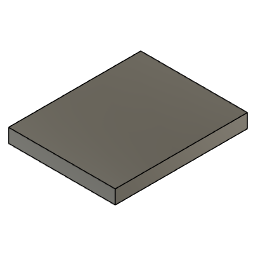
Mold Design Day#20 v4 (Autodesk Fusion 360 design; units mm, degrees)
Autodesk Fusion 360 part; units mm, degrees
box "BoxPrimitive1" add length 50 width 35 height 3 placed x (0, 1, 0) y (-1, 0, 0) z (0, 0, 1) at (35, 0, 0) makes body 1 in component "Keychaing"
fillet "Fillet1" radius 7 4 edges at (35, 0, 1.5) (0, 0, 1.5) (0, 50, 1.5) (35, 50, 1.5) on bodies 1 in component "Keychaing"
sketch "Sketch2" plane through (0, 0, 3) normal (0, 0, 1) x (-1, 0, 0) in component "Keychaing"
  arc A0 (-35, -43) -> (-28, -50) centre (-28, -43) ccw
  line L0 (-28, -50) -> (-7, -50)
  arc A1 (-7, -50) -> (0, -43) centre (-7, -43) ccw
  line L1 (0, -43) -> (0, -7)
  arc A2 (0, -7) -> (-7, 0) centre (-7, -7) ccw
  line L2 (-7, 0) -> (-28, 0)
  arc A3 (-28, 0) -> (-35, -7) centre (-28, -7) ccw
  line L3 (-35, -7) -> (-35, -43)
  line L4 (-17.5, -50) -> (-17.5, -45)
  dimension "d8" = 5
  constraint vertical L4
  constraint midpoint L0 L4.start
  measures "d8" distance of L4.start L4.end
hole "Hole1" at (17.5, 45, 3) direction (0, 0, -1) diameter 5 depth 3 tip angle 180 bodies 1 in component "Keychaing"
sketch "Sketch3" plane through (0, 0, 3) normal (0, 0, 1) x (-1, 0, 0) in component "Keychaing"
  circle A0 centre (-17.5, -45) radius 2.5
  arc A1 (-35, -43) -> (-28, -50) centre (-28, -43) ccw
  line L0 (-28, -50) -> (-7, -50)
  arc A2 (-7, -50) -> (0, -43) centre (-7, -43) ccw
  line L1 (0, -43) -> (0, -7)
  arc A3 (0, -7) -> (-7, 0) centre (-7, -7) ccw
  line L2 (-7, 0) -> (-28, 0)
  arc A4 (-28, 0) -> (-35, -7) centre (-28, -7) ccw
  line L3 (-35, -7) -> (-35, -43)
  spline S0 degree 3 poles (-7.2465, -28.2329) (-7.1727, -28.1591) (-7.1727, -22.1159) (-7.2465, -22.0421) knots 0 0 0 0 1 1 1 1
  spline S1 degree 3 poles (-7.2465, -22.0421) (-7.3203, -21.9683) (-8.9136, -21.9683) (-8.9614, -22.0465) knots 0 0 0 0 1 1 1 1
  spline S2 degree 3 poles (-8.9614, -22.0465) (-8.9787, -22.0725) (-9.0048, -22.6543) (-9.0178, -23.3358) knots 0 0 0 0 1 1 1 1
  line L4 (-9.0178, -23.3358) -> (-9.0395, -24.5731)
  line L5 (-9.0395, -24.5731) -> (-9.5561, -23.3575)
  spline S3 degree 3 poles (-9.5561, -23.3575) (-9.8383, -22.689) (-10.0988, -22.1072) (-10.1379, -22.0682) knots 0 0 0 0 1 1 1 1
  spline S4 degree 3 poles (-10.1379, -22.0682) (-10.1943, -21.9987) (-10.2985, -21.99) (-11.0409, -21.99) knots 0 0 0 0 1 1 1 1
  spline S5 degree 3 poles (-11.0409, -21.99) (-11.8744, -21.99) (-11.8831, -21.99) (-11.9482, -22.0942) knots 0 0 0 0 1 1 1 1
  spline S6 degree 3 poles (-11.9482, -22.0942) (-12.009, -22.181) (-12.0133, -22.5501) (-12.0046, -25.1983) knots 0 0 0 0 1 1 1 1
  spline S7 degree 3 poles (-12.0046, -25.1983) (-11.9916, -27.8118) (-11.9829, -28.2068) (-11.9265, -28.2416) knots 0 0 0 0 1 1 1 1
  spline S8 degree 3 poles (-11.9265, -28.2416) (-11.8223, -28.3067) (-10.2464, -28.298) (-10.203, -28.2329) knots 0 0 0 0 1 1 1 1
  spline S9 degree 3 poles (-10.203, -28.2329) (-10.1856, -28.2025) (-10.1596, -27.6207) (-10.1465, -26.9435) knots 0 0 0 0 1 1 1 1
  line L6 (-10.1465, -26.9435) -> (-10.1248, -25.7149)
  line L7 (-10.1248, -25.7149) -> (-9.5865, -26.9739)
  spline S10 degree 3 poles (-9.5865, -26.9739) (-9.2913, -27.6685) (-9.0221, -28.2459) (-8.9874, -28.2589) knots 0 0 0 0 1 1 1 1
  spline S11 degree 3 poles (-8.9874, -28.2589) (-8.8528, -28.311) (-7.2986, -28.285) (-7.2465, -28.2329) knots 0 0 0 0 1 1 1 1
  spline S12 degree 3 poles (-9.5171, -26.6092) (-10.0901, -25.2634) (-10.1683, -25.1115) (-10.2507, -25.1245) knots 0 0 0 0 1 1 1 1
  spline S13 degree 3 poles (-10.2507, -25.1245) (-10.3419, -25.1375) (-10.3419, -25.1418) (-10.3549, -26.6266) knots 0 0 0 0 1 1 1 1
  line L8 (-10.3549, -26.6266) -> (-10.3636, -28.1113)
  line L9 (-10.3636, -28.1113) -> (-11.0799, -28.1113)
  line L10 (-11.0799, -28.1113) -> (-11.7963, -28.1113)
  line L11 (-11.7963, -28.1113) -> (-11.7876, -25.1505)
  line L12 (-11.7876, -25.1505) -> (-11.7746, -22.1854)
  line L13 (-11.7746, -22.1854) -> (-11.0539, -22.1724)
  spline S14 degree 3 poles (-11.0539, -22.1724) (-10.5112, -22.1637) (-10.3202, -22.1767) (-10.2855, -22.2158) knots 0 0 0 0 1 1 1 1
  spline S15 degree 3 poles (-10.2855, -22.2158) (-10.2594, -22.2462) (-10.0424, -22.7411) (-9.7992, -23.3141) knots 0 0 0 0 1 1 1 1
  spline S16 degree 3 poles (-9.7992, -23.3141) (-9.0135, -25.1766) (-9.0178, -25.1635) (-8.9136, -25.1505) knots 0 0 0 0 1 1 1 1
  spline S17 degree 3 poles (-8.9136, -25.1505) (-8.8224, -25.1375) (-8.8224, -25.1288) (-8.8094, -23.6484) knots 0 0 0 0 1 1 1 1
  line L14 (-8.8094, -23.6484) -> (-8.8007, -22.1637)
  line L15 (-8.8007, -22.1637) -> (-8.0931, -22.1724)
  line L16 (-8.0931, -22.1724) -> (-7.3898, -22.1854)
  line L17 (-7.3898, -22.1854) -> (-7.3768, -25.0941)
  spline S18 degree 3 poles (-7.3768, -25.0941) (-7.3724, -26.696) (-7.3768, -28.0288) (-7.3898, -28.0592) knots 0 0 0 0 1 1 1 1
  spline S19 degree 3 poles (-7.3898, -28.0592) (-7.4028, -28.0983) (-7.5938, -28.1113) (-8.1452, -28.1113) knots 0 0 0 0 1 1 1 1
  line L18 (-8.1452, -28.1113) -> (-8.8789, -28.1113)
  line L19 (-8.8789, -28.1113) -> (-9.5171, -26.6092)
  spline S20 degree 3 poles (-13.8454, -28.2112) (-13.8237, -28.1678) (-13.446, -26.7872) (-13.0118, -25.1418) knots 0 0 0 0 1 1 1 1
  spline S21 degree 3 poles (-13.0118, -25.1418) (-12.4127, -22.8974) (-12.2261, -22.1333) (-12.2608, -22.0812) knots 0 0 0 0 1 1 1 1
  spline S22 degree 3 poles (-12.2608, -22.0812) (-12.2999, -22.0204) (-12.4214, -22.0117) (-13.1898, -22.0117) knots 0 0 0 0 1 1 1 1
  line L20 (-13.1898, -22.0117) -> (-14.0711, -22.0117)
  line L21 (-14.0711, -22.0117) -> (-14.1276, -22.1637)
  spline S23 degree 3 poles (-14.1276, -22.1637) (-14.1536, -22.2462) (-14.2014, -22.4285) (-14.2274, -22.5674) knots 0 0 0 0 1 1 1 1
  line L22 (-14.2274, -22.5674) -> (-14.2795, -22.8192)
  line L23 (-14.2795, -22.8192) -> (-14.8916, -22.8062)
  line L24 (-14.8916, -22.8062) -> (-15.5038, -22.7932)
  line L25 (-15.5038, -22.7932) -> (-15.5819, -22.4502)
  spline S24 degree 3 poles (-15.5819, -22.4502) (-15.6253, -22.2592) (-15.6818, -22.0812) (-15.7122, -22.0465) knots 0 0 0 0 1 1 1 1
  spline S25 degree 3 poles (-15.7122, -22.0465) (-15.7469, -21.9987) (-15.9379, -21.99) (-16.6282, -21.9987) knots 0 0 0 0 1 1 1 1
  spline S26 degree 3 poles (-16.6282, -21.9987) (-17.3836, -22.0117) (-17.5008, -22.0204) (-17.5399, -22.0855) knots 0 0 0 0 1 1 1 1
  spline S27 degree 3 poles (-17.5399, -22.0855) (-17.5746, -22.1376) (-17.4009, -22.867) (-16.7931, -25.1679) knots 0 0 0 0 1 1 1 1
  spline S28 degree 3 poles (-16.7931, -25.1679) (-16.3547, -26.8219) (-15.977, -28.2025) (-15.9553, -28.2329) knots 0 0 0 0 1 1 1 1
  spline S29 degree 3 poles (-15.9553, -28.2329) (-15.9205, -28.2719) (-15.6557, -28.285) (-14.896, -28.285) knots 0 0 0 0 1 1 1 1
  spline S30 degree 3 poles (-14.896, -28.285) (-13.9756, -28.285) (-13.8801, -28.2763) (-13.8454, -28.2112) knots 0 0 0 0 1 1 1 1
  spline S31 degree 3 poles (-16.5544, -25.2504) (-16.9668, -23.6918) (-17.3184, -22.359) (-17.3315, -22.2896) knots 0 0 0 0 1 1 1 1
  line L26 (-17.3315, -22.2896) -> (-17.3619, -22.1637)
  line L27 (-17.3619, -22.1637) -> (-16.6499, -22.1637)
  spline S32 degree 3 poles (-16.6499, -22.1637) (-16.2592, -22.1637) (-15.9205, -22.181) (-15.8945, -22.1984) knots 0 0 0 0 1 1 1 1
  spline S33 degree 3 poles (-15.8945, -22.1984) (-15.8684, -22.2158) (-15.8207, -22.3373) (-15.7946, -22.4676) knots 0 0 0 0 1 1 1 1
  spline S34 degree 3 poles (-15.7946, -22.4676) (-15.7642, -22.5978) (-15.7208, -22.7715) (-15.6948, -22.8496) knots 0 0 0 0 1 1 1 1
  line L28 (-15.6948, -22.8496) -> (-15.6514, -22.9885)
  line L29 (-15.6514, -22.9885) -> (-14.9003, -22.9885)
  spline S35 degree 3 poles (-14.9003, -22.9885) (-14.0364, -22.9885) (-14.1015, -23.0233) (-14.0103, -22.5544) knots 0 0 0 0 1 1 1 1
  spline S36 degree 3 poles (-14.0103, -22.5544) (-13.98, -22.3981) (-13.9365, -22.2462) (-13.9105, -22.2201) knots 0 0 0 0 1 1 1 1
  spline S37 degree 3 poles (-13.9105, -22.2201) (-13.8801, -22.1767) (-13.6761, -22.1637) (-13.1551, -22.1637) knots 0 0 0 0 1 1 1 1
  line L30 (-13.1551, -22.1637) -> (-12.4388, -22.1637)
  line L31 (-12.4388, -22.1637) -> (-12.4692, -22.2852)
  spline S38 degree 3 poles (-12.4692, -22.2852) (-12.5126, -22.4719) (-13.9669, -27.9507) (-13.993, -28.0375) knots 0 0 0 0 1 1 1 1
  spline S39 degree 3 poles (-13.993, -28.0375) (-14.0147, -28.107) (-14.0885, -28.1113) (-14.9133, -28.1026) knots 0 0 0 0 1 1 1 1
  line L32 (-14.9133, -28.1026) -> (-15.8077, -28.0896)
  line L33 (-15.8077, -28.0896) -> (-16.5544, -25.2504)
  spline S40 degree 3 poles (-14.7961, -26.1447) (-14.731, -26.0622) (-14.3403, -24.2215) (-14.375, -24.139) knots 0 0 0 0 1 1 1 1
  spline S41 degree 3 poles (-14.375, -24.139) (-14.4097, -24.0391) (-15.3475, -24.0435) (-15.3866, -24.1433) knots 0 0 0 0 1 1 1 1
  spline S42 degree 3 poles (-15.3866, -24.1433) (-15.4169, -24.2215) (-15.0696, -25.9276) (-14.9915, -26.0796) knots 0 0 0 0 1 1 1 1
  spline S43 degree 3 poles (-14.9915, -26.0796) (-14.9307, -26.1968) (-14.8612, -26.2228) (-14.7961, -26.1447) knots 0 0 0 0 1 1 1 1
  spline S44 degree 3 poles (-15.1825, -24.304) (-15.1825, -24.2432) (-14.6398, -24.2215) (-14.6051, -24.2823) knots 0 0 0 0 1 1 1 1
  spline S45 degree 3 poles (-14.6051, -24.2823) (-14.5834, -24.3126) (-14.8135, -25.4674) (-14.8656, -25.5933) knots 0 0 0 0 1 1 1 1
  spline S46 degree 3 poles (-14.8656, -25.5933) (-14.8873, -25.6498) (-15.1782, -24.4646) (-15.1825, -24.304) knots 0 0 0 0 1 1 1 1
  spline S47 degree 3 poles (-17.8828, -28.2329) (-17.809, -28.1591) (-17.809, -22.1159) (-17.8828, -22.0421) knots 0 0 0 0 1 1 1 1
  spline S48 degree 3 poles (-17.8828, -22.0421) (-17.9219, -22.0031) (-18.2866, -21.99) (-19.259, -21.99) knots 0 0 0 0 1 1 1 1
  spline S49 degree 3 poles (-19.259, -21.99) (-20.7481, -21.9944) (-20.9044, -22.0161) (-21.4254, -22.2766) knots 0 0 0 0 1 1 1 1
  spline S50 degree 3 poles (-21.4254, -22.2766) (-21.7857, -22.4589) (-22.0028, -22.6803) (-22.1677, -23.0276) knots 0 0 0 0 1 1 1 1
  spline S51 degree 3 poles (-22.1677, -23.0276) (-22.2719, -23.249) (-22.2806, -23.3185) (-22.2806, -23.8134) knots 0 0 0 0 1 1 1 1
  spline S52 degree 3 poles (-22.2806, -23.8134) (-22.2806, -24.317) (-22.2719, -24.3734) (-22.159, -24.6165) knots 0 0 0 0 1 1 1 1
  spline S53 degree 3 poles (-22.159, -24.6165) (-22.0939, -24.7598) (-21.9593, -24.9595) (-21.8595, -25.0594) knots 0 0 0 0 1 1 1 1
  line L34 (-21.8595, -25.0594) -> (-21.6815, -25.2417)
  line L35 (-21.6815, -25.2417) -> (-21.8595, -25.4414)
  spline S54 degree 3 poles (-21.8595, -25.4414) (-22.3761, -26.0275) (-22.3153, -27.1996) (-21.7423, -27.7553) knots 0 0 0 0 1 1 1 1
  spline S55 degree 3 poles (-21.7423, -27.7553) (-21.5252, -27.9637) (-21.1605, -28.1417) (-20.7915, -28.2242) knots 0 0 0 0 1 1 1 1
  spline S56 degree 3 poles (-20.7915, -28.2242) (-20.4051, -28.3023) (-17.961, -28.311) (-17.8828, -28.2329) knots 0 0 0 0 1 1 1 1
  spline S57 degree 3 poles (-20.8393, -28.0115) (-21.6164, -27.7857) (-21.955, -27.3776) (-21.9897, -26.6092) knots 0 0 0 0 1 1 1 1
  spline S58 degree 3 poles (-21.9897, -26.6092) (-22.0158, -26.0709) (-21.9333, -25.8278) (-21.6164, -25.4978) knots 0 0 0 0 1 1 1 1
  line L36 (-21.6164, -25.4978) -> (-21.3819, -25.2504)
  line L37 (-21.3819, -25.2504) -> (-21.6164, -25.0159)
  spline S59 degree 3 poles (-21.6164, -25.0159) (-21.8899, -24.7468) (-22.0201, -24.4993) (-22.0896, -24.1346) knots 0 0 0 0 1 1 1 1
  spline S60 degree 3 poles (-22.0896, -24.1346) (-22.2285, -23.3966) (-21.9203, -22.7367) (-21.2951, -22.4372) knots 0 0 0 0 1 1 1 1
  spline S61 degree 3 poles (-21.2951, -22.4372) (-20.8176, -22.2071) (-20.6613, -22.1854) (-19.2851, -22.1854) knots 0 0 0 0 1 1 1 1
  line L38 (-19.2851, -22.1854) -> (-18.0261, -22.1854)
  line L39 (-18.0261, -22.1854) -> (-18.0131, -25.1505)
  line L40 (-18.0131, -25.1505) -> (-18.0044, -28.12)
  line L41 (-18.0044, -28.12) -> (-19.2938, -28.0983)
  spline S62 degree 3 poles (-19.2938, -28.0983) (-20.3183, -28.0853) (-20.6396, -28.0679) (-20.8393, -28.0115) knots 0 0 0 0 1 1 1 1
  spline S63 degree 3 poles (-19.5021, -26.8436) (-19.4891, -26.8089) (-19.4848, -26.5484) (-19.4891, -26.2619) knots 0 0 0 0 1 1 1 1
  line L42 (-19.4891, -26.2619) -> (-19.5021, -25.7453)
  line L43 (-19.5021, -25.7453) -> (-19.8147, -25.7323)
  spline S64 degree 3 poles (-19.8147, -25.7323) (-20.327, -25.7106) (-20.5527, -25.8625) (-20.5962, -26.2619) knots 0 0 0 0 1 1 1 1
  spline S65 degree 3 poles (-20.5962, -26.2619) (-20.6222, -26.479) (-20.531, -26.7134) (-20.3834, -26.8046) knots 0 0 0 0 1 1 1 1
  spline S66 degree 3 poles (-20.3834, -26.8046) (-20.2402, -26.8957) (-19.5325, -26.9261) (-19.5021, -26.8436) knots 0 0 0 0 1 1 1 1
  spline S67 degree 3 poles (-20.3053, -26.5832) (-20.3617, -26.518) (-20.3921, -26.4312) (-20.3921, -26.3053) knots 0 0 0 0 1 1 1 1
  spline S68 degree 3 poles (-20.3921, -26.3053) (-20.3921, -26.0448) (-20.2532, -25.9406) (-19.9102, -25.9406) knots 0 0 0 0 1 1 1 1
  line L44 (-19.9102, -25.9406) -> (-19.6541, -25.9406)
  line L45 (-19.6541, -25.9406) -> (-19.6541, -26.3097)
  line L46 (-19.6541, -26.3097) -> (-19.6541, -26.6787)
  line L47 (-19.6541, -26.6787) -> (-19.9363, -26.6787)
  spline S69 degree 3 poles (-19.9363, -26.6787) (-20.1664, -26.6787) (-20.2315, -26.6613) (-20.3053, -26.5832) knots 0 0 0 0 1 1 1 1
  spline S70 degree 3 poles (-19.5325, -24.6469) (-19.4935, -24.6165) (-19.4804, -24.4603) (-19.4891, -24.0044) knots 0 0 0 0 1 1 1 1
  line L48 (-19.4891, -24.0044) -> (-19.5021, -23.401)
  line L49 (-19.5021, -23.401) -> (-19.806, -23.3879)
  spline S71 degree 3 poles (-19.806, -23.3879) (-20.1924, -23.3706) (-20.3965, -23.4314) (-20.5441, -23.605) knots 0 0 0 0 1 1 1 1
  spline S72 degree 3 poles (-20.5441, -23.605) (-20.6526, -23.7309) (-20.6613, -23.77) (-20.6439, -24.0565) knots 0 0 0 0 1 1 1 1
  spline S73 degree 3 poles (-20.6439, -24.0565) (-20.6266, -24.4038) (-20.5614, -24.521) (-20.3183, -24.6209) knots 0 0 0 0 1 1 1 1
  spline S74 degree 3 poles (-20.3183, -24.6209) (-20.1664, -24.686) (-19.6237, -24.7034) (-19.5325, -24.6469) knots 0 0 0 0 1 1 1 1
  spline S75 degree 3 poles (-20.3357, -24.3604) (-20.4399, -24.2692) (-20.4572, -24.2215) (-20.4572, -24.0305) knots 0 0 0 0 1 1 1 1
  spline S76 degree 3 poles (-20.4572, -24.0305) (-20.4572, -23.8394) (-20.4399, -23.7917) (-20.3357, -23.7005) knots 0 0 0 0 1 1 1 1
  spline S77 degree 3 poles (-20.3357, -23.7005) (-20.2358, -23.6137) (-20.1664, -23.5963) (-19.9319, -23.5963) knots 0 0 0 0 1 1 1 1
  line L50 (-19.9319, -23.5963) -> (-19.6541, -23.5963)
  line L51 (-19.6541, -23.5963) -> (-19.6541, -24.0305)
  line L52 (-19.6541, -24.0305) -> (-19.6541, -24.4646)
  line L53 (-19.6541, -24.4646) -> (-19.9319, -24.4646)
  spline S78 degree 3 poles (-19.9319, -24.4646) (-20.1664, -24.4646) (-20.2358, -24.4472) (-20.3357, -24.3604) knots 0 0 0 0 1 1 1 1
  spline S79 degree 3 poles (-22.7017, -28.2329) (-22.6279, -28.1591) (-22.6279, -22.1159) (-22.7017, -22.0421) knots 0 0 0 0 1 1 1 1
  spline S80 degree 3 poles (-22.7017, -22.0421) (-22.7364, -22.0074) (-22.9926, -21.99) (-23.5613, -21.99) knots 0 0 0 0 1 1 1 1
  spline S81 degree 3 poles (-23.5613, -21.99) (-24.13, -21.99) (-24.3862, -22.0074) (-24.4209, -22.0421) knots 0 0 0 0 1 1 1 1
  spline S82 degree 3 poles (-24.4209, -22.0421) (-24.4947, -22.1159) (-24.4947, -28.1591) (-24.4209, -28.2329) knots 0 0 0 0 1 1 1 1
  spline S83 degree 3 poles (-24.4209, -28.2329) (-24.3471, -28.3067) (-22.7755, -28.3067) (-22.7017, -28.2329) knots 0 0 0 0 1 1 1 1
  line L54 (-24.2559, -25.1375) -> (-24.2559, -22.1637)
  line L55 (-24.2559, -22.1637) -> (-23.5526, -22.1724)
  line L56 (-23.5526, -22.1724) -> (-22.845, -22.1854)
  line L57 (-22.845, -22.1854) -> (-22.832, -25.0941)
  spline S84 degree 3 poles (-22.832, -25.0941) (-22.8276, -26.696) (-22.832, -28.0288) (-22.845, -28.0592) knots 0 0 0 0 1 1 1 1
  spline S85 degree 3 poles (-22.845, -28.0592) (-22.858, -28.0983) (-23.0447, -28.1113) (-23.5613, -28.1113) knots 0 0 0 0 1 1 1 1
  line L58 (-23.5613, -28.1113) -> (-24.2559, -28.1113)
  line L59 (-24.2559, -28.1113) -> (-24.2559, -25.1375)
  spline S86 degree 3 poles (-24.9158, -28.2329) (-24.842, -28.1591) (-24.842, -22.1159) (-24.9158, -22.0421) knots 0 0 0 0 1 1 1 1
  spline S87 degree 3 poles (-24.9158, -22.0421) (-24.9549, -22.0031) (-25.4715, -21.99) (-26.9779, -21.99) knots 0 0 0 0 1 1 1 1
  spline S88 degree 3 poles (-26.9779, -21.99) (-28.9185, -21.99) (-28.988, -21.9944) (-29.0314, -22.0725) knots 0 0 0 0 1 1 1 1
  spline S89 degree 3 poles (-29.0314, -22.0725) (-29.0531, -22.1203) (-29.0748, -22.4415) (-29.0748, -22.8105) knots 0 0 0 0 1 1 1 1
  spline S90 degree 3 poles (-29.0748, -22.8105) (-29.0748, -23.4357) (-29.0705, -23.4661) (-28.9793, -23.5269) knots 0 0 0 0 1 1 1 1
  spline S91 degree 3 poles (-28.9793, -23.5269) (-28.8968, -23.5876) (-28.7058, -23.5963) (-27.7854, -23.5963) knots 0 0 0 0 1 1 1 1
  line L60 (-27.7854, -23.5963) -> (-26.6871, -23.5963)
  line L61 (-26.6871, -23.5963) -> (-26.6871, -25.8886)
  spline S92 degree 3 poles (-26.6871, -25.8886) (-26.6871, -27.6121) (-26.674, -28.1938) (-26.635, -28.2329) knots 0 0 0 0 1 1 1 1
  spline S93 degree 3 poles (-26.635, -28.2329) (-26.5612, -28.3067) (-24.9896, -28.3067) (-24.9158, -28.2329) knots 0 0 0 0 1 1 1 1
  line L62 (-26.5134, -25.7453) -> (-26.5351, -23.401)
  line L63 (-26.5351, -23.401) -> (-27.6986, -23.3879)
  line L64 (-27.6986, -23.3879) -> (-28.8577, -23.3793)
  line L65 (-28.8577, -23.3793) -> (-28.8577, -22.7715)
  line L66 (-28.8577, -22.7715) -> (-28.8577, -22.1637)
  line L67 (-28.8577, -22.1637) -> (-26.9606, -22.1724)
  line L68 (-26.9606, -22.1724) -> (-25.0591, -22.1854)
  line L69 (-25.0591, -22.1854) -> (-25.046, -25.1505)
  line L70 (-25.046, -25.1505) -> (-25.0374, -28.1113)
  line L71 (-25.0374, -28.1113) -> (-25.7624, -28.1026)
  line L72 (-25.7624, -28.1026) -> (-26.4917, -28.0896)
  line L73 (-26.4917, -28.0896) -> (-26.5134, -25.7453)
extrude "Extrude1" add sketch "Sketch3" along normal blind 1 contours S12 S13 L8 L9 L10 L11 L12 L13 S14 S15 S16 S17 L14 L15 L16 L17 S18 S19 L18 L19 | S31 L26 L27 S32 S33 S34 L28 L29 S35 S36 S37 L30 L31 S38 S39 L32 L33 | S57 S58 L36 L37 S59 S60 S61 L38 L39 L40 L41 S62 | L54 L55 L56 L57 S84 S85 L58 L59 | L62 L63 L64 L65 L66 L67 L68 L69 L70 L71 L72 L73 bodies 1 in component "Keychaing"
box "BoxPrimitive2" add length 57 width 46 height 6 placed x (0, -1, 0) y (1, 0, 0) z (0, 0, 1) at (-5, 53, 0) separate body makes body 2 in component "Keychaing"
combine "Combine1" operation cut target body 2 tool bodies 1 keep tools result as body 3 in component "Component"
draft "Draft1" angle 3 neutral plane through (-5, 53, 0) pull (0, 0, -1) 8 faces at (35, 19, 1) (34.9921, 43.3331, 1) (21, 50, 1) (0.0079, 43.3331, 1) (0, 19, 1) (0.0079, 6.6669, 1) (21, 0, 1) (32.3271, 1.4976, 1) on bodies 3 in component "Component"
draft "Draft2" angle 3 neutral plane through (-5, 53, 0) pull (0, 0, -1) 1 faces at (17.6246, 42.5031, 2) on bodies 3 in component "Component"
component "Keychaing" placed x (1, 0, 0) y (0, 1, 0) z (0, 0, 1) at (0, 0, 0)
component "Component" placed x (1, 0, 0) y (0, 1, 0) z (0, 0, 1) at (0, 0, 0)
named bodies: "Keychain", "Mold"
